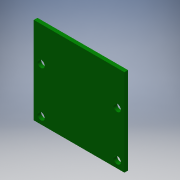
# Autodesk Inventor part: kamera
Saved by Autodesk Inventor 2016 (Build 200138000, 138)
## iProperties
Created: 2015-01-29
Part Number: kamera
Material: Generic
Document SubType Name: Modeling
Designer: Kuba
Density: 5.09076 g/cm^3
Appearance: Default
Mass: 4 g
Surface Area: 14.3367 cm^2
Volume: 0.785737 cm^3
Author: Kuba
Autodesk Inventor part; units mm, degrees
ref_plane "YZ Plane" through (0, 0, 0) normal (1, 0, 0) x (0, 1, 0)
ref_plane "XZ Plane" through (0, 0, 0) normal (0, 1, 0) x (-1, 0, 0)
ref_plane "XY Plane" through (0, 0, 0) normal (0, 0, 1) x (1, 0, 0)
sketch "Sketch1" plane through (0, 0, 0) normal (0, 1, 0) x (-1, 0, 0)
  line L0 (12.5, 12) -> (-12.5, 12)
  line L1 (-12.5, 12) -> (-12.5, -12)
  line L2 (-12.5, -12) -> (12.5, -12)
  line L3 (12.5, -12) -> (12.5, 12)
  line L4 (12.5, 12) -> (-12.5, -12) construction
  line L5 (-12.5, 12) -> (12.5, -12) construction
  point P0 (0, 0)
  dimension "d0" = 25
  dimension "d1" = 24
  constraints: 12 end point, 2 midpoint, 2 parallel, 1 horizontal, 1 perpendicular
  measures "d0" distance of L2.end L1.end
  measures "d1" distance of L1.end L0.end
extrude "Extrusion1" add sketch "Sketch1" along normal blind 1
sketch "Sketch2" plane through (0, 1, 0) normal (0, 1, 0) x (1, 0, 0)
  line L0 (-12.5, 12) -> (-10.5, 12)
  line L1 (-10.5, 12) -> (-10.5, 10)
  line L2 (-10.5, 10) -> (-12.5, 10)
  line L3 (-12.5, 10) -> (-12.5, 12)
  line L4 (12.5, 12) -> (10.5, 12)
  line L5 (10.5, 12) -> (10.5, 10)
  line L6 (10.5, 10) -> (12.5, 10)
  line L7 (12.5, 10) -> (12.5, 12)
  line L8 (-12.5, 12) -> (-10.5, 12)
  line L9 (-10.5, 12) -> (-10.5, -2.5)
  line L10 (-10.5, -2.5) -> (-12.5, -2.5)
  line L11 (-12.5, -2.5) -> (-12.5, 12)
  line L12 (12.5, 12) -> (10.5, 12)
  line L13 (10.5, 12) -> (10.5, -2.5)
  line L14 (10.5, -2.5) -> (12.5, -2.5)
  line L15 (12.5, -2.5) -> (12.5, 12)
  circle A0 centre (-10.5, 10) radius 1
  circle A1 centre (-10.5, -2.5) radius 1
  circle A2 centre (10.5, -2.5) radius 1
  circle A3 centre (10.5, 10) radius 1
  point P0 (0, 0)
  dimension "d4" = 2
  dimension "d5" = 2
  dimension "d6" = 2
  dimension "d7" = 2
  dimension "d8" = 14.5
  dimension "d9" = 14.5
  dimension "d10" = 2
  dimension "d11" = 2
  dimension "d12" = 2
  dimension "d13" = 2
  constraints: 32 end point, 8 parallel, 4 centre point, 4 coincident, 4 horizontal, 4 perpendicular
  measures "d4" distance of L1.end L2.end
  measures "d5" distance of L0.end L1.end
  measures "d6" distance of L6.end L5.end
  measures "d7" distance of L5.end L4.end
  measures "d8" distance of L8.end L9.end
  measures "d9" distance of L13.end L12.end
  measures "d10" diameter of A0
  measures "d11" diameter of A1
  measures "d12" diameter of A2
  measures "d13" diameter of A3
extrude "Extrusion2" cut sketch "Sketch2" against normal up to next contours A0 L9 L1 | L1 L2 A0 | L2 L9 A0 | A1 L9 L10 | L10 L9 A1 | A3 L6 L5 | L5 L13 A3 | A3 L13 L6 | A2 L13 L14 | L14 L13 A2
sketch "Sketch3" plane through (0, 1, 0) normal (0, 1, 0) x (1, 0, 0)
  circle A0 centre (-10.5, -2.5) radius 1 projected
  circle A1 centre (10.5, -2.5) radius 1 projected
  line L0 (-12.5, 12) -> (-12.5, -12) projected
  line L1 (-10.5, -2.5) -> (10.5, -2.5)
  line L2 (-4, -6.5) -> (4, -6.5)
  line L3 (4, -6.5) -> (4, 1.5)
  line L4 (4, 1.5) -> (-4, 1.5)
  line L5 (-4, 1.5) -> (-4, -6.5)
  line L6 (-4, -6.5) -> (4, 1.5) construction
  line L7 (4, -6.5) -> (-4, 1.5) construction
  point P0 (0, 0)
  point P1 (0, -2.5)
  dimension "d16" = 8
  dimension "d17" = 8
  constraints: 14 end point, 3 midpoint, 2 parallel, 2 perpendicular, 1 horizontal
  measures "d16" distance of L4.end L3.end
  measures "d17" distance of L3.end L2.end
extrude "Extrusion3" add sketch "Sketch3" along normal blind 1 contours L5 L4 L3 L1 | L1 L3 L2 L5
sketch "Sketch4" plane through (0, 2, 0) normal (0, 1, 0) x (1, 0, 0)
  line L0 (-4, 1.5) -> (4, -6.5)
  circle A0 centre (0, -2.5) radius 3.5
  point P0 (0, 0)
  dimension "d20" = 7
  constraints: 2 end point, 1 centre point, 1 midpoint
  measures "d20" diameter of A0
extrude "Extrusion4" add sketch "Sketch4" along normal blind 4
sketch "Sketch5" plane through (0, 6, 2.5) normal (0, 1, 0) x (1, 0, 0)
  circle A0 centre (0, 0) radius 3.5 projected
  circle A1 centre (0, 0) radius 2.5
  point P0 (0, 2.5)
  dimension "d23" = 5
  constraints: 1 centre point, 1 coincident
  measures "d23" diameter of A1
extrude "Extrusion5" cut sketch "Sketch5" against normal blind 1 contours A1
body "Solid1"
